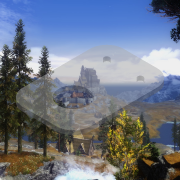
# Autodesk Inventor part: C33_TK_IdiotLightBracket
Saved by Autodesk Inventor 2015 SP1 (Build 190203100, 203)
## iProperties
Created: 2016-02-06
Part Number: C33_TK_IdiotLightBracket
Material: Polycarbonate, Clear
Document SubType Name: Modeling
Designer: TheeTimatahee
Density: 1.2 g/cm^3
Appearance: Polycarbonate - Clear
Author: TheeTimatahee
Autodesk Inventor part; units mm, degrees
ref_plane "YZ Plane" through (0, 0, 0) normal (1, 0, 0) x (0, 1, 0)
ref_plane "XZ Plane" through (0, 0, 0) normal (0, 1, 0) x (-1, 0, 0)
ref_plane "XY Plane" through (0, 0, 0) normal (0, 0, 1) x (1, 0, 0)
sketch "Sketch1" plane through (0, 0, 0) normal (0, 0, 1) x (1, 0, 0)
  line L0 (-25.4, -1.5875) -> (25.4, -1.5875)
  line L1 (25.4, -1.5875) -> (25.4, 1.5875)
  line L2 (25.4, 1.5875) -> (-25.4, 1.5875)
  line L3 (-25.4, 1.5875) -> (-25.4, -1.5875)
  line L4 (-25.4, -1.5875) -> (25.4, 1.5875) construction
  line L5 (25.4, -1.5875) -> (-25.4, 1.5875) construction
  point P0 (0, 0)
  dimension "d0" = 3.175
  dimension "d1" = 50.8
  constraints: 12 end point, 2 midpoint, 2 parallel, 1 horizontal, 1 perpendicular
  measures "d0" distance of L0.end L1.end
  measures "d1" distance of L1.end L2.end
extrude "Extrusion1" add sketch "Sketch1" along normal blind 76.2
sketch "Sketch2" plane through (-25.4, 1.5875, 0) normal (0, 1, 0) x (1, 0, 0)
  line L0 (50.8, 0) -> (50.8, -76.2) projected
  line L1 (0, 0) -> (0, -76.2) projected
  line L2 (50.8, 0) -> (0, 0) projected
  line L3 (50.8, -76.2) -> (0, -76.2) projected
  point P0 (25.4, 0)
  point P1 (38.1, -12.7)
  point P2 (12.7, -12.7)
  point P3 (25.4, -50.8)
  dimension "d4" = 12.7
  dimension "d5" = 12.7
  dimension "d6" = 12.7
  dimension "d7" = 12.7
  dimension "d8" = 25.4
  dimension "d9" = 25.4
  measures "d4" distance from line of L0 point (38.1, -12.7)
  measures "d5" distance from line of L1 point (12.7, -12.7)
  measures "d6" distance from line of L2 point (12.7, -12.7)
  measures "d7" distance from line of L2 point (38.1, -12.7)
  measures "d8" distance from line of L0 point (25.4, -50.8)
  measures "d9" distance from line of point (25.4, -50.8) L3
hole "Hole1" at (12.7, 1.5875, 12.7) at (-12.7, 1.5875, 12.7) direction (0, -1, 0) diameter 4.1402 end through all
hole "Hole2" at (0, 1.5875, 50.8) direction (0, -1, 0) diameter 22 end through all
fillet "Fillet1" radius 12.7 4 edges at (-25.4, 0, 0) (25.4, 0, 0) (25.4, 0, 76.2) (-25.4, 0, 76.2)
body "Solid1"
